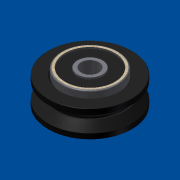
# Autodesk Inventor part: MSK01-05A
Saved by Autodesk Inventor 2013 (Build 170138000, 138)
## iProperties
Created: 2012-01-26
Part Number: MSK01-05A
Document SubType Name: Modeling
Designer: ERF
Density: 1 g/cm^3
Description: v-wheel assembly
Material: Generic
Mass: 3.44894 g
Surface Area: 40.6852 cm^2
Volume: 2.44224 cm^3
Stock Number: B30037
Vendor: buildlog.net
Project: Shapeoko
Author: ERF
Title: V-Wheel Assembly
Autodesk Inventor part; units mm, degrees
ref_plane "YZ Plane" through (0, 0, 0) normal (1, 0, 0) x (0, 1, 0)
ref_plane "XZ Plane" through (0, 0, 0) normal (0, 1, 0) x (-1, 0, 0)
ref_plane "XY Plane" through (0, 0, 0) normal (0, 0, 1) x (1, 0, 0)
sketch "Sketch1" plane through (0, 5.5, 0) normal (0, 1, 0) x (1, 0, 0)
  circle A0 centre (0, 0) radius 7.615 projected
  circle A1 centre (0, 0) radius 7 projected
extrude "Extrusion1" add sketch "Sketch1" along normal blind 0.00254
sketch "Sketch2" plane through (0, -5.5, 0) normal (0, -1, 0) x (1, 0, 0)
  circle A0 centre (0, 0) radius 7.615 projected
  circle A1 centre (0, 0) radius 7 projected
extrude "Extrusion2" add sketch "Sketch2" along normal blind 0.00254
body "Solid1"
body "Srf1"
